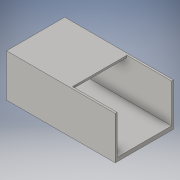
# Autodesk Inventor part: RTCcase
Saved by Autodesk Inventor 2016 (Build 200138000, 138)
## iProperties
Created: 2017-03-30
Part Number: RTCcase
Material: Generic
Document SubType Name: Modeling
Designer: Jorian Bruslind
Density: 1 g/cm^3
Appearance: Default
Author: Jorian Bruslind
Autodesk Inventor part; units mm, degrees
ref_plane "YZ Plane" through (0, 0, 0) normal (1, 0, 0) x (0, 1, 0)
ref_plane "XZ Plane" through (0, 0, 0) normal (0, 1, 0) x (-1, 0, 0)
ref_plane "XY Plane" through (0, 0, 0) normal (0, 0, 1) x (1, 0, 0)
sketch "Sketch1" plane through (0, 0, 0) normal (0, 1, 0) x (-1, 0, 0)
  line L0 (0, 0) -> (44.45, 0)
  line L1 (44.45, 0) -> (44.45, -23.8125)
  line L2 (44.45, -23.8125) -> (0, -23.8125)
  line L3 (0, -23.8125) -> (0, 0)
  dimension "d0" = 44.45
  dimension "d1" = 23.8125
  constraints: 8 end point, 2 parallel, 1 horizontal, 1 perpendicular
  measures "d0" distance of L1.end L2.end
  measures "d1" distance of L0.end L1.end
extrude "Extrusion1" add sketch "Sketch1" along normal blind 1.5875
sketch "Sketch2" plane through (0, 1.5875, 0) normal (0, 1, 0) x (1, 0, 0)
  line L0 (-44.45, 0) -> (0, 0) projected
  line L1 (0, 0) -> (0, 0.7937)
  line L2 (0, 0.7937) -> (-0.7938, 0.7937)
  line L3 (-44.45, 23.8125) -> (-44.45, 0) projected
  line L4 (-44.45, 23.8125) -> (-44.45, 23.0187)
  line L5 (-44.45, 23.0187) -> (-43.6563, 23.0187)
  line L6 (-0.7938, 0.7937) -> (-43.6563, 0.7937)
  line L7 (-43.6563, 0.7937) -> (-43.6563, 23.0187)
  line L8 (-43.6563, 23.0187) -> (-0.7938, 23.0187)
  line L9 (-44.45, 23.8125) -> (0, 23.8125)
  line L10 (0, 0) -> (-44.45, 0)
  line L11 (-44.45, 0) -> (-44.45, 23.8125)
  line L12 (-0.7938, 23.0187) -> (0, 23.0187)
  line L13 (0, 0) -> (0, 23.8125) projected
  line L14 (0, 23.0187) -> (0, 23.8125)
  dimension "d4" = 0.7937
  dimension "d5" = 0.7937
  dimension "d6" = 0.7937
  dimension "d7" = 0.7937
  constraints: 24 end point, 4 horizontal, 2 parallel, 2 perpendicular, 1 collinear, 1 point on line
  measures "d4" distance of L0.end L1.end
  measures "d5" distance of L1.end L2.end
  measures "d6" distance of L3.start L4.end
  measures "d7" distance of L4.end L5.end
extrude "Extrusion3" add sketch "Sketch2" along normal blind 15.875 contours L3 L5 L7 L6 L2 L1 L0 | L3 L9 L13 L12 L8 L5
sketch "Sketch3" plane through (-43.6563, 1.5875, -0.7937) normal (1, 0, 0) x (0, 0, -1)
  line L0 (0, 15.875) -> (22.225, 15.875) projected
  line L1 (22.225, 15.875) -> (0, 15.875)
  line L2 (0, 15.875) -> (0, 15.0876)
  line L3 (0, 15.0876) -> (22.225, 15.0876)
  line L4 (22.225, 15.0876) -> (22.225, 15.875)
  point P0 (-0.7937, -1.5875)
  dimension "d12" = 0.7874
  constraints: 8 end point, 2 parallel, 1 horizontal, 1 perpendicular
  measures "d12" distance of L2.end L1.end
extrude "Extrusion4" add sketch "Sketch3" along normal blind 25.4
body "Solid1"
